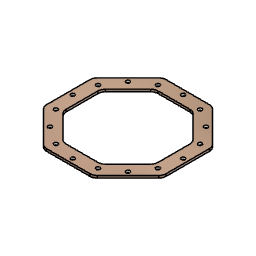
stage 2 connector clamp v5 (Autodesk Fusion 360 design; units mm, degrees)
Autodesk Fusion 360 part; units mm, degrees
note: some values were not read from the file. Set by a fixed rule: the direction of a hole.
sketch "Sketch1" plane through (0, 0, 0) normal (0, 1, 0) x (1, 0, 0)
  circle A0 centre (0, 0) radius 60 construction
  line L0 (-65, -26.9239) -> (-26.9239, -65)
  line L1 (-26.9239, -65) -> (26.9239, -65)
  line L2 (26.9239, -65) -> (65, -26.9239)
  line L3 (65, -26.9239) -> (65, 26.9239)
  line L4 (65, 26.9239) -> (26.9239, 65)
  line L5 (26.9239, 65) -> (-26.9239, 65)
  line L6 (-26.9239, 65) -> (-65, 26.9239)
  line L7 (-65, 26.9239) -> (-65, -26.9239)
  line L8 (-20.7107, -50) -> (20.7107, -50)
  line L9 (20.7107, -50) -> (50, -20.7107)
  line L10 (50, -20.7107) -> (50, 20.7107)
  line L11 (50, 20.7107) -> (20.7107, 50)
  line L12 (20.7107, 50) -> (-20.7107, 50)
  line L13 (-20.7107, 50) -> (-50, 20.7107)
  line L14 (-50, 20.7107) -> (-50, -20.7107)
  line L15 (-50, -20.7107) -> (-20.7107, -50)
  point P0 (-60, 0)
  dimension "d1" = 120
  dimension "d2" = 65
  dimension "d3" = 130
  dimension "d4" = -15
  constraint coincident A0.centre origin
  constraint coincident A0 P0
  constraint horizontal A0.centre P0
  constraint horizontal L5
  measures "d1" diameter of A0
  measures "d2" distance of A0.centre L7
  measures "d3" distance of L3 L7 A0.centre
extrude "Extrude1" add sketch "Sketch1" along normal blind 2.5
hole "Hole1" at (-60, 0, 0) direction (0, 1, 0) diameter 4.234 depth 100 tip angle 118
thread "Thread1" "ISO Metric profile 5.0 M5x0.8 6H" thread offset 0 thread depth 10
pattern_circular "C-Pattern1" count 16 over 360 about axis through (0, 1.75, 0) along (0, 1, 0) of "Hole1"
fillet "Fillet1" radius 8 16 edges at (-26.9239, 1.25, 65) (26.9239, 1.25, 65) (65, 1.25, 26.9239) (65, 1.25, -26.9239) (26.9239, 1.25, -65) (-26.9239, 1.25, -65) (-65, 1.25, -26.9239) (-65, 1.25, 26.9239) (20.7107, 1.25, -50) (50, 1.25, -20.7107) (50, 1.25, 20.7107) (20.7107, 1.25, 50) (-20.7107, 1.25, 50) (-50, 1.25, 20.7107) (-50, 1.25, -20.7107) (-20.7107, 1.25, -50)
sketch "stage 2 connector clamp cutting pattern" plane through (0, 2.5, 0) normal (0, 1, 0) x (-1, 0, 0)
  arc A0 (65, 23.6102) -> (62.6569, 29.267) centre (57, 23.6102) ccw
  line L0 (62.6569, 29.267) -> (29.267, 62.6569)
  arc A1 (29.267, 62.6569) -> (23.6102, 65) centre (23.6102, 57) ccw
  line L1 (23.6102, 65) -> (-23.6102, 65)
  arc A2 (-23.6102, 65) -> (-29.267, 62.6569) centre (-23.6102, 57) ccw
  line L2 (-29.267, 62.6569) -> (-62.6569, 29.267)
  arc A3 (-62.6569, 29.267) -> (-65, 23.6102) centre (-57, 23.6102) ccw
  line L3 (-65, 23.6102) -> (-65, -23.6102)
  arc A4 (-65, -23.6102) -> (-62.6569, -29.267) centre (-57, -23.6102) ccw
  line L4 (-62.6569, -29.267) -> (-29.267, -62.6569)
  arc A5 (-29.267, -62.6569) -> (-23.6102, -65) centre (-23.6102, -57) ccw
  line L5 (-23.6102, -65) -> (23.6102, -65)
  arc A6 (23.6102, -65) -> (29.267, -62.6569) centre (23.6102, -57) ccw
  line L6 (29.267, -62.6569) -> (62.6569, -29.267)
  arc A7 (62.6569, -29.267) -> (65, -23.6102) centre (57, -23.6102) ccw
  line L7 (65, -23.6102) -> (65, 23.6102)
  circle A8 centre (55.4328, -22.961) radius 2.117
  circle A9 centre (42.4264, -42.4264) radius 2.117
  circle A10 centre (22.961, -55.4328) radius 2.117
  circle A11 centre (0, -60) radius 2.117
  circle A12 centre (-22.961, -55.4328) radius 2.117
  circle A13 centre (-42.4264, -42.4264) radius 2.117
  circle A14 centre (-55.4328, -22.961) radius 2.117
  circle A15 centre (-60, 0) radius 2.117
  circle A16 centre (-55.4328, 22.961) radius 2.117
  circle A17 centre (-42.4264, 42.4264) radius 2.117
  circle A18 centre (-22.961, 55.4328) radius 2.117
  circle A19 centre (0, 60) radius 2.117
  circle A20 centre (22.961, 55.4328) radius 2.117
  circle A21 centre (42.4264, 42.4264) radius 2.117
  circle A22 centre (55.4328, 22.961) radius 2.117
  circle A23 centre (60, 0) radius 2.117
  line L8 (23.0538, 47.6569) -> (47.6569, 23.0538)
  arc A24 (50, 17.397) -> (47.6569, 23.0538) centre (42, 17.397) ccw
  line L9 (50, 17.397) -> (50, -17.397)
  arc A25 (47.6569, -23.0538) -> (50, -17.397) centre (42, -17.397) ccw
  line L10 (47.6569, -23.0538) -> (23.0538, -47.6569)
  arc A26 (17.397, -50) -> (23.0538, -47.6569) centre (17.397, -42) ccw
  line L11 (17.397, -50) -> (-17.397, -50)
  arc A27 (-23.0538, -47.6569) -> (-17.397, -50) centre (-17.397, -42) ccw
  line L12 (-23.0538, -47.6569) -> (-47.6569, -23.0538)
  arc A28 (-50, -17.397) -> (-47.6569, -23.0538) centre (-42, -17.397) ccw
  line L13 (-50, -17.397) -> (-50, 17.397)
  arc A29 (-47.6569, 23.0538) -> (-50, 17.397) centre (-42, 17.397) ccw
  line L14 (-47.6569, 23.0538) -> (-23.0538, 47.6569)
  arc A30 (-17.397, 50) -> (-23.0538, 47.6569) centre (-17.397, 42) ccw
  line L15 (-17.397, 50) -> (17.397, 50)
  arc A31 (23.0538, 47.6569) -> (17.397, 50) centre (17.397, 42) ccw
